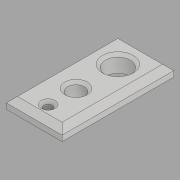
# Autodesk Inventor part: 2-2-1
Saved by Autodesk Inventor 2019 (Build 230136000, 136)
## iProperties
Created: 2020-11-06
Part Number: 2-2-1
Material: 一般
Document SubType Name: Modeling
Designer: Sugar
Density: 1 g/cm^3
Appearance: 預設
Author: Sugar
Autodesk Inventor part; units mm, degrees
ref_plane "YZ Plane" through (0, 0, 0) normal (1, 0, 0) x (0, 1, 0)
ref_plane "XZ Plane" through (0, 0, 0) normal (0, 1, 0) x (-1, 0, 0)
ref_plane "XY Plane" through (0, 0, 0) normal (0, 0, 1) x (1, 0, 0)
sketch "草圖1" plane through (0, 0, 0) normal (0, 1, 0) x (-1, 0, 0)
  line L0 (100, -50) -> (-100, -50)
  line L1 (-100, -50) -> (-100, 50)
  line L2 (-100, 50) -> (100, 50)
  line L3 (100, 50) -> (100, -50)
  point P0 (0, 0)
  point P1 (0, -50)
  point P2 (-100, 0)
  dimension "d0" = 100
  dimension "d1" = 200
  constraints: 8 end point, 2 midpoint, 2 parallel, 1 horizontal, 1 horizontal alignment, 1 perpendicular, 1 vertical alignment
  measures "d0" distance of L0.end L1.end
  measures "d1" distance of L1.end L2.end
extrude "擠出1" add sketch "草圖1" along normal blind 30
chamfer "倒角1" distance 10 angle 45 8 edges at (0, 30, 50) (0, 0, 50) (-100, 30, 0) (-100, 0, 0) (0, 30, -50) (100, 30, 0) (100, 0, 0) (0, 0, -50)
sketch "草圖2" plane through (0, 30, 0) normal (0, 1, 0) x (1, 0, 0)
  line L0 (-100, 50) -> (-100, -50) projected
  circle A0 centre (-75, 0) radius 7.5
  circle A1 centre (-25, 0) radius 15
  circle A2 centre (50, 0) radius 22.5
  point P0 (0, 0)
  point P1 (-100, 0)
  dimension "d7" = 15
  dimension "d8" = 30
  dimension "d9" = 45
  dimension "d10" = 25
  dimension "d11" = 75
  dimension "d12" = 75
  constraints: 3 centre point, 3 horizontal alignment, 1 midpoint
  measures "d7" diameter of A0
  measures "d8" diameter of A1
  measures "d9" diameter of A2
  measures "d10" distance from line of L0 A0.centre
  measures "d11" distance from line of L0 A1.centre
  measures "d12" distance of A1.centre A2.centre
extrude "擠出2" cut sketch "草圖2" against normal through all
chamfer "倒角2" distance 5 angle 45 3 edges at (-82.5, 30, 0) (-40, 30, 0) (27.5, 30, 0)
